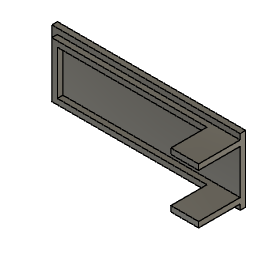
usb-lid v2 (Autodesk Fusion 360 design; units mm, degrees)
Autodesk Fusion 360 part; units mm, degrees
sketch "Sketch1" plane through (0, 0, 0) normal (0, 1, 0) x (1, 0, 0)
  line L0 (0, 0) -> (-68, 0)
  line L1 (-68, 0) -> (-68, -24)
  line L2 (-68, -24) -> (0, -24)
  line L3 (0, -24) -> (0, 0)
  constraint horizontal L0
  constraint vertical L1
  constraint horizontal L2
  constraint vertical L3
  constraint coincident L0.start L3.end
extrude "Extrude1" add sketch "Sketch1" along normal blind 2
sketch "Sketch2" plane through (0, 0, 0) normal (0, 1, 0) x (1, 0, 0)
  line L0 (-66, -22) -> (0, -22)
  line L1 (0, -22) -> (0, -20)
  line L2 (0, -20) -> (-66, -20)
  line L3 (-66, -20) -> (-66, -22)
  constraint horizontal L0
  constraint vertical L1
  constraint horizontal L2
  constraint vertical L3
extrude "Extrude2" add sketch "Sketch2" against normal blind 2
sketch "Sketch3" plane through (0, 0, 0) normal (0, 1, 0) x (1, 0, 0)
  line L0 (-66, -20) -> (-64, -20)
  line L1 (-64, -20) -> (-64, -2)
  line L2 (-64, -2) -> (-66, -2)
  line L3 (-66, -2) -> (-66, -20)
  constraint horizontal L0
  constraint vertical L1
  constraint horizontal L2
  constraint vertical L3
extrude "Extrude3" add sketch "Sketch3" against normal blind 2
sketch "Sketch4" plane through (0, 0, 0) normal (0, 1, 0) x (1, 0, 0)
  line L0 (-64, -4) -> (0, -4)
  line L1 (0, -4) -> (0, -2)
  line L2 (0, -2) -> (-64, -2)
  line L3 (-64, -2) -> (-64, -4)
  constraint horizontal L0
  constraint vertical L1
  constraint horizontal L2
  constraint vertical L3
extrude "Extrude4" add sketch "Sketch4" against normal blind 2
sketch "Sketch5" plane through (0, 0, 0) normal (0, 1, 0) x (1, 0, 0)
  line L0 (-10, -22) -> (0, -22)
  line L1 (0, -22) -> (0, -20)
  line L2 (0, -20) -> (-10, -20)
  line L3 (-10, -20) -> (-10, -22)
  constraint horizontal L0
  constraint vertical L1
  constraint horizontal L2
  constraint vertical L3
extrude "Extrude5" add sketch "Sketch5" against normal blind 10
extrude "Extrude6" add 1 faces at (-6.6667, -10, 20.6667) along direction (0, -1, 0) blind 5
sketch "Sketch6" plane through (0, 0, 0) normal (0, 1, 0) x (1, 0, 0)
  line L0 (-10, -4) -> (0, -4)
  line L1 (0, -4) -> (0, -2)
  line L2 (0, -2) -> (-10, -2)
  line L3 (-10, -2) -> (-10, -4)
  constraint horizontal L0
  constraint vertical L1
  constraint horizontal L2
  constraint vertical L3
extrude "Extrude7" add sketch "Sketch6" against normal blind 15
